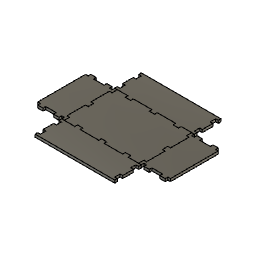
3D_Box (Autodesk Fusion 360 design; units mm, degrees)
Autodesk Fusion 360 part; units mm, degrees
sketch "Sketch1" plane through (0, 0, 0) normal (0, 0, 1) x (1, 0, 0)
  line L0 (0, 100) -> (150, 100)
  line L1 (150, 100) -> (150, 0)
  line L2 (150, 0) -> (0, 0)
  line L3 (0, 0) -> (0, 100)
  line L4 (145, 0) -> (145, 10)
  line L5 (145, 10) -> (150, 10)
  line L6 (150, 10) -> (150, 45)
  line L7 (150, 45) -> (145, 45)
  line L8 (145, 45) -> (145, 55)
  line L9 (145, 55) -> (150, 55)
  line L10 (150, 55) -> (150, 90)
  line L11 (150, 90) -> (145, 90)
  line L12 (145, 90) -> (145, 100)
  line L13 (145, 100) -> (150, 100)
  line L14 (145, 0) -> (150, 0)
  line L15 (75, 100) -> (75, 0) construction
  line L16 (5, 90) -> (5, 100)
  line L17 (0, 90) -> (5, 90)
  line L18 (5, 55) -> (0, 55)
  line L19 (5, 45) -> (5, 55)
  line L20 (0, 45) -> (5, 45)
  line L21 (5, 10) -> (0, 10)
  line L22 (5, 0) -> (5, 10)
  line L23 (25, 100) -> (25, 95)
  line L24 (25, 95) -> (35, 95)
  line L25 (35, 95) -> (35, 100)
  line L26 (35, 100) -> (70, 100)
  line L27 (70, 100) -> (70, 95)
  line L28 (70, 95) -> (80, 95)
  line L29 (80, 95) -> (80, 100)
  line L30 (80, 100) -> (115, 100)
  line L31 (115, 100) -> (115, 95)
  line L32 (115, 95) -> (125, 95)
  line L33 (125, 95) -> (125, 100)
  line L34 (125, 100) -> (145, 100)
  line L35 (25, 100) -> (5, 100)
  line L36 (5, 50) -> (145, 50) construction
  line L37 (25, 0) -> (25, 5)
  line L38 (35, 5) -> (35, 0)
  line L39 (25, 5) -> (35, 5)
  line L40 (70, 0) -> (70, 5)
  line L41 (70, 5) -> (80, 5)
  line L42 (80, 5) -> (80, 0)
  line L43 (115, 0) -> (115, 5)
  line L44 (115, 5) -> (125, 5)
  line L45 (125, 5) -> (125, 0)
  dimension "d1" = 150
  dimension "d2" = 100
  dimension "d5" = 5
  dimension "d6" = 5
  dimension "d7" = 5
  dimension "d8" = 5
  dimension "d9" = 5
  dimension "d10" = 5
  dimension "d11" = 10
  dimension "d12" = 10
  dimension "d13" = 10
  dimension "d14" = 100
  dimension "d15" = 140
  dimension "d16" = 5
  dimension "d17" = 5
  dimension "d18" = 5
  dimension "d19" = 5
  dimension "d20" = 5
  dimension "d21" = 5
  dimension "d22" = 10
  dimension "d23" = 10
  dimension "d24" = 10
  dimension "d25" = 20
  dimension "d26" = 20
  constraint horizontal L0
  constraint vertical L1
  constraint horizontal L2
  constraint vertical L3
  constraint coincident L2.end L3.start
  constraint vertical L4
  constraint perpendicular L4 L5
  constraint perpendicular L5 L6
  constraint perpendicular L4 L7
  constraint perpendicular L5 L8
  constraint perpendicular L8 L9
  constraint perpendicular L5 L10
  constraint perpendicular L8 L11
  constraint perpendicular L5 L12
  constraint perpendicular L12 L13
  constraint perpendicular L4 L14
  constraint equal L6 L10
  constraint coincident L1.end L2.start
  constraint midpoint L0 L15.start
  constraint midpoint L2 L15.end
  constraint symmetric L4.start L15 L22.start
  constraint symmetric L4.end L15 L21.start
  constraint symmetric L5.end L15 L21.end
  constraint symmetric L6.end L15 L20.start
  constraint symmetric L7.end L15 L19.start
  constraint symmetric L8.end L15 L18.start
  constraint symmetric L9.end L15 L18.end
  constraint symmetric L10.end L15 L17.start
  constraint symmetric L11.end L15 L16.start
  constraint symmetric L12.end L15 L16.end
  constraint vertical L23
  constraint perpendicular L23 L24
  constraint perpendicular L24 L25
  constraint perpendicular L25 L26
  constraint perpendicular L26 L27
  constraint perpendicular L25 L28
  constraint perpendicular L28 L29
  constraint perpendicular L29 L30
  constraint perpendicular L30 L31
  constraint perpendicular L29 L32
  constraint perpendicular L30 L33
  constraint perpendicular L33 L34
  constraint perpendicular L23 L35
  constraint equal L26 L30
  constraint coincident L16.end L35.end
  constraint midpoint L19 L36.start
  constraint midpoint L8 L36.end
  constraint symmetric L23.start L36 L37.start
  constraint symmetric L23.end L36 L37.end
  constraint symmetric L24.end L36 L38.start
  constraint symmetric L25.end L36 L38.end
  constraint symmetric L26.end L36 L40.start
  constraint symmetric L27.end L36 L40.end
  constraint symmetric L28.end L36 L41.end
  constraint symmetric L29.end L36 L42.end
  constraint symmetric L30.end L36 L43.start
  constraint symmetric L31.end L36 L43.end
  constraint symmetric L32.end L36 L44.end
  constraint symmetric L33.end L36 L45.end
  measures "d1" distance of L1 L3
  measures "d2" distance of L0 L2
  measures "d5" distance of L12.end L0.end
  measures "d6" distance of L10.end L11.end
  measures "d7" distance of L8.end L9.end
  measures "d8" distance of L6.end L7.end
  measures "d9" distance of L4.end L5.end
  measures "d10" distance of L4.start L1.end
  measures "d11" distance of L11.end L12.end
  measures "d12" distance of L7.end L8.end
  measures "d13" distance of L4.start L4.end
  measures "d14" distance of L4.start L12.end
  measures "d15" horizontal distance of L12.end L16.end
  measures "d16" distance of L23.start L23.end
  measures "d17" distance of L24.end L25.end
  measures "d18" distance of L26.end L27.end
  measures "d19" distance of L28.end L29.end
  measures "d20" distance of L30.end L31.end
  measures "d21" distance of L32.end L33.end
  measures "d22" distance of L23 L25
  measures "d23" distance of L27.end L28.end
  measures "d24" distance of L31.end L32.end
  measures "d25" distance of L23.start L16.end
  measures "d26" distance of L33.end L12.end
extrude "Extrude1" add sketch "Sketch1" along normal blind 5 contours L0 L1 L2 L3 L4 L5 L6 L7 L8 L9 L10 L11 L12 L16 L17 L18 L19 L20 L21 L22 L23 L24 L25 L26 L27 L28 L29 L30 L31 L32 L33 L34 L35 L37 L38 L39 L40 L41 L42 L43 L44 L45 makes body 1
sketch "Sketch1 (2)" plane through (0, 0, 0) normal (0, 0, 1) x (1, 0, 0) in component "sSide"
  line L0 (115, 0) -> (115, 5)
  line L1 (115, 5) -> (125, 5)
  line L2 (125, 5) -> (125, 0)
  line L3 (125, 0) -> (145, 0)
  line L4 (145, 0) -> (145, 10)
  line L5 (145, 10) -> (150, 10)
  line L6 (150, 10) -> (150, 45)
  line L7 (150, 45) -> (145, 45)
  line L8 (145, 45) -> (145, 55)
  line L9 (145, 55) -> (150, 55)
  line L10 (150, 55) -> (150, 90)
  line L11 (150, 90) -> (145, 90)
  line L12 (145, 90) -> (145, 100)
  line L13 (145, 100) -> (125, 100)
  line L14 (125, 100) -> (125, 95)
  line L15 (125, 95) -> (115, 95)
  line L16 (115, 95) -> (115, 100)
  line L17 (115, 100) -> (80, 100)
  line L18 (80, 100) -> (80, 95)
  line L19 (80, 95) -> (70, 95)
  line L20 (70, 95) -> (70, 100)
  line L21 (70, 100) -> (35, 100)
  line L22 (35, 100) -> (35, 95)
  line L23 (35, 95) -> (25, 95)
  line L24 (25, 95) -> (25, 100)
  line L25 (25, 100) -> (5, 100)
  line L26 (5, 100) -> (5, 90)
  line L27 (5, 90) -> (0, 90)
  line L28 (0, 90) -> (0, 55)
  line L29 (0, 55) -> (5, 55)
  line L30 (5, 55) -> (5, 45)
  line L31 (5, 45) -> (0, 45)
  line L32 (0, 45) -> (0, 10)
  line L33 (0, 10) -> (5, 10)
  line L34 (5, 10) -> (5, 0)
  line L35 (5, 0) -> (25, 0)
  line L36 (25, 0) -> (25, 5)
  line L37 (25, 5) -> (35, 5)
  line L38 (35, 5) -> (35, 0)
  line L39 (35, 0) -> (70, 0)
  line L40 (70, 0) -> (70, 5)
  line L41 (70, 5) -> (80, 5)
  line L42 (80, 5) -> (80, 0)
  line L43 (80, 0) -> (115, 0)
  line L44 (145, 100) -> (200, 100)
  line L45 (200, 100) -> (200, 0)
  line L46 (200, 0) -> (145, 0)
  line L47 (150, 95) -> (155, 95)
  line L48 (155, 95) -> (155, 100)
  line L49 (155, 100) -> (165, 100)
  line L50 (165, 100) -> (165, 95)
  line L51 (165, 95) -> (185, 95)
  line L52 (185, 95) -> (185, 100)
  line L53 (185, 100) -> (195, 100)
  line L54 (195, 100) -> (195, 95)
  line L55 (195, 95) -> (200, 95)
  line L56 (150, 95) -> (150, 100)
  line L57 (150, 100) -> (145, 100)
  line L58 (200, 50) -> (145, 50) construction
  line L59 (150, 5) -> (150, 0)
  line L60 (155, 5) -> (155, 0)
  line L61 (150, 5) -> (155, 5)
  line L62 (165, 0) -> (165, 5)
  line L63 (165, 5) -> (185, 5)
  line L64 (185, 5) -> (185, 0)
  line L65 (195, 0) -> (195, 5)
  line L66 (195, 5) -> (200, 5)
  dimension "d28" = 50
  dimension "d43" = 10
  dimension "d44" = 10
  dimension "d45" = 5
  dimension "d46" = 50
  dimension "d47" = 5
  dimension "d48" = 5
  dimension "d49" = 5
  dimension "d50" = 5
  dimension "d52" = 5
  dimension "d53" = 5
  constraint coincident L12.end L13.start
  constraint perpendicular L12 L44
  constraint perpendicular L44 L45
  constraint coincident L3.end L4.start
  constraint perpendicular L4 L46
  constraint horizontal L47
  constraint perpendicular L47 L48
  constraint perpendicular L48 L49
  constraint perpendicular L49 L50
  constraint perpendicular L50 L51
  constraint perpendicular L49 L52
  constraint perpendicular L52 L53
  constraint perpendicular L53 L54
  constraint perpendicular L54 L55
  constraint equal L47 L55
  constraint perpendicular L47 L56
  constraint perpendicular L56 L57
  constraint midpoint L45 L58.start
  constraint midpoint L8 L58.end
  constraint symmetric L47.start L58 L59.start
  constraint symmetric L47.end L58 L60.start
  constraint symmetric L48.end L58 L60.end
  constraint symmetric L49.end L58 L62.start
  constraint symmetric L50.end L58 L62.end
  constraint symmetric L51.end L58 L63.end
  constraint symmetric L52.end L58 L64.end
  constraint symmetric L53.end L58 L65.start
  constraint symmetric L54.end L58 L65.end
  constraint symmetric L55.end L58 L66.end
  constraint symmetric L56.end L58 L59.end
  measures "d28" horizontal distance of L10.end L44.end
  measures "d43" distance of L48 L50
  measures "d44" distance of L52 L54
  measures "d45" distance of L47.start L47.end
  measures "d46" distance of L47.start L55.end
  measures "d47" distance of L47.end L48.end
  measures "d48" distance of L49.end L50.end
  measures "d49" distance of L51.end L52.end
  measures "d50" distance of L53.end L54.end
  measures "d52" distance of L47.start L56.end
  measures "d53" distance of L56.end L12.end
extrude "Extrude1'" add sketch "Sketch1 (2)" along normal blind 5 separate body contours L4 L5 L6 L7 L8 L9 L10 L11 L12 L44 L45 L46 L47 L48 L49 L50 L51 L52 L53 L54 L55 L56 L57 L59 L60 L61 L62 L63 L64 L65 L66 makes body 2 in component "sSide"
sketch "Sketch1 (3)" plane through (0, 0, 0) normal (0, 0, 1) x (1, 0, 0) in component "lSide"
  line L0 (115, 0) -> (115, 5)
  line L1 (115, 5) -> (125, 5)
  line L2 (125, 5) -> (125, 0)
  line L3 (125, 0) -> (145, 0)
  line L4 (145, 0) -> (145, 10)
  line L5 (145, 10) -> (150, 10)
  line L6 (150, 10) -> (150, 45)
  line L7 (150, 45) -> (145, 45)
  line L8 (145, 45) -> (145, 55)
  line L9 (145, 55) -> (150, 55)
  line L10 (150, 55) -> (150, 90)
  line L11 (150, 90) -> (145, 90)
  line L12 (145, 90) -> (145, 100)
  line L13 (145, 100) -> (125, 100)
  line L14 (125, 100) -> (125, 95)
  line L15 (125, 95) -> (115, 95)
  line L16 (115, 95) -> (115, 100)
  line L17 (115, 100) -> (80, 100)
  line L18 (80, 100) -> (80, 95)
  line L19 (80, 95) -> (70, 95)
  line L20 (70, 95) -> (70, 100)
  line L21 (70, 100) -> (35, 100)
  line L22 (35, 100) -> (35, 95)
  line L23 (35, 95) -> (25, 95)
  line L24 (25, 95) -> (25, 100)
  line L25 (25, 100) -> (5, 100)
  line L26 (5, 100) -> (5, 90)
  line L27 (5, 90) -> (0, 90)
  line L28 (0, 90) -> (0, 55)
  line L29 (0, 55) -> (5, 55)
  line L30 (5, 55) -> (5, 45)
  line L31 (5, 45) -> (0, 45)
  line L32 (0, 45) -> (0, 10)
  line L33 (0, 10) -> (5, 10)
  line L34 (5, 10) -> (5, 0)
  line L35 (5, 0) -> (25, 0)
  line L36 (25, 0) -> (25, 5)
  line L37 (25, 5) -> (35, 5)
  line L38 (35, 5) -> (35, 0)
  line L39 (35, 0) -> (70, 0)
  line L40 (70, 0) -> (70, 5)
  line L41 (70, 5) -> (80, 5)
  line L42 (80, 5) -> (80, 0)
  line L43 (80, 0) -> (115, 0)
  line L44 (145, 100) -> (150, 100)
  line L45 (150, 100) -> (150, 150)
  line L46 (150, 150) -> (0, 150)
  line L47 (0, 150) -> (0, 100)
  line L48 (5, 100) -> (0, 100)
  line L49 (150, 150) -> (150, 145)
  line L50 (150, 145) -> (145, 145)
  line L51 (145, 145) -> (145, 135)
  line L52 (145, 135) -> (150, 135)
  line L53 (145, 115) -> (150, 115)
  line L54 (150, 115) -> (150, 135)
  line L55 (145, 115) -> (145, 105)
  line L56 (145, 105) -> (150, 105)
  line L57 (150, 105) -> (150, 100)
  line L58 (75, 150) -> (75, 95) construction
  line L59 (0, 145) -> (5, 145)
  line L60 (5, 145) -> (5, 135)
  line L61 (5, 135) -> (0, 135)
  line L62 (5, 115) -> (0, 115)
  line L63 (5, 115) -> (5, 105)
  line L64 (5, 105) -> (0, 105)
  dimension "d31" = 50
  dimension "d32" = 150
  dimension "d33" = 5
  dimension "d34" = 10
  dimension "d35" = 10
  dimension "d36" = 5
  dimension "d37" = 5
  dimension "d38" = 5
  dimension "d39" = 50
  dimension "d40" = 5
  constraint coincident L12.end L13.start
  constraint perpendicular L12 L44
  constraint perpendicular L44 L45
  constraint perpendicular L28 L46
  constraint perpendicular L27 L47
  constraint coincident L25.end L26.start
  constraint perpendicular L47 L48
  constraint equal L44 L48
  constraint vertical L49
  constraint perpendicular L49 L50
  constraint perpendicular L50 L51
  constraint perpendicular L51 L52
  constraint parallel L52 L53
  constraint perpendicular L52 L54
  constraint perpendicular L53 L55
  constraint perpendicular L55 L56
  constraint perpendicular L53 L57
  constraint equal L49 L57
  constraint coincident L45.end L46.start
  constraint midpoint L46 L58.start
  constraint midpoint L19 L58.end
  constraint symmetric L49.end L58 L59.start
  constraint symmetric L50.end L58 L59.end
  constraint symmetric L51.end L58 L60.end
  constraint symmetric L52.end L58 L61.end
  constraint symmetric L53.start L58 L62.start
  constraint symmetric L53.end L58 L62.end
  constraint symmetric L55.end L58 L63.end
  constraint symmetric L56.end L58 L64.end
  measures "d31" distance of L13 L46
  measures "d32" distance of L45 L47
  measures "d33" distance of L49.end L50.end
  measures "d34" distance of L50.end L51.end
  measures "d35" distance of L53.start L55.end
  measures "d36" distance of L51.end L52.end
  measures "d37" distance of L53.start L53.end
  measures "d38" distance of L55.end L56.end
  measures "d39" distance of L45.end L44.end
  measures "d40" distance of L56.end L44.end
extrude "Extrude2" add sketch "Sketch1 (3)" along normal blind 5 separate body contours L13 L14 L15 L16 L17 L18 L19 L20 L21 L22 L23 L24 L25 L44 L45 L46 L47 L48 L49 L50 L51 L52 L53 L54 L55 L56 L57 L59 L60 L61 L62 L63 L64 makes body 3
copy_body "CopyPasteBodies1" bodies 3 makes body 4
move_body "Move1" bodies 4 to x (1, 0, 0) y (0, 1, 0) z (0, 0, 1) at (0, -150, 0)
move_body "Move2" bodies 4 to x (-1, 0, 0) y (0, -1, 0) z (0, 0, 1) at (0, 0, 0)
move_body "Move3" bodies 4 to x (1, 0, 0) y (0, 1, 0) z (0, 0, 1) at (150, -50, 0)
copy_body "CopyPasteBodies2" bodies 2 makes body 5
move_body "Move4" bodies 5 to x (1, 0, 0) y (0, 1, 0) z (0, 0, 1) at (-240, 0, 0)
move_body "Move5" bodies 5 to x (-1, 0, 0) y (0, -1, 0) z (0, 0, 1) at (0, 0, 0)
move_body "Move6" bodies 5 to x (1, 0, 0) y (0, 1, 0) z (0, 0, 1) at (-90, 100, 0)
copy_body "CutPasteBodies1" bodies 5 removing the originals makes body 6 in component "sSide"
copy_body "CutPasteBodies1'" bodies 3 removing the originals makes body 7 in component "lSide"
copy_body "CutPasteBodies2" bodies 4 removing the originals makes body 8 in component "lSide"
component "sSide" placed x (1, 0, 0) y (0, 1, 0) z (0, 0, 1) at (0, 0, 0)
component "lSide" placed x (1, 0, 0) y (0, 1, 0) z (0, 0, 1) at (0, 0, 0)
equation "d6 = d5"
equation "d7 = d6"
equation "d8 = d5"
equation "d9 = d8"
equation "d10 = d9"
equation "d16 = d5"
equation "d17 = d5"
equation "d18 = d5"
equation "d19 = d5"
equation "d20 = d5"
equation "d21 = d5"
equation "d22 = d11"
equation "d23 = d11"
equation "d24 = d11"
equation "d35 = d34"
equation "d36 = d33"
equation "d37 = d33"
equation "d38 = d33"
equation "d44 = d43"
equation "d48 = d47"
equation "d49 = d47"
equation "d50 = d47"
equation "d52 = d47"
equation "d53 = d47"
named bodies: "bottom"
